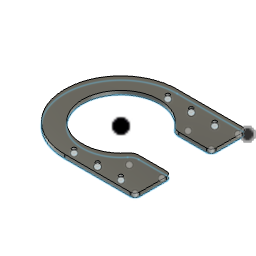
Base (Autodesk Fusion 360 design; units mm, degrees)
Autodesk Fusion 360 part; units mm, degrees
note: some values were not read from the file. Set by a fixed rule: which sketch regions a step uses.
sketch "草图1" plane through (0, 0, 0) normal (0, 0, 1) x (1, 0, 0)
  line L0 (0, 60) -> (70, 60)
  line L1 (75, 55) -> (75, 40)
  line L2 (75, -40) -> (75, -55)
  line L3 (70, -60) -> (0, -60)
  arc A0 (0, 60) -> (0, -60) centre (0, 0) ccw
  circle A1 centre (0, -50) radius 2.1 construction
  circle A2 centre (25, -50) radius 2.1 construction
  circle A3 centre (50, -50) radius 2.1 construction
  circle A4 centre (0, 50) radius 2.1 construction
  circle A5 centre (25, 50) radius 2.1 construction
  circle A6 centre (50, 50) radius 2.1 construction
  circle A7 centre (50, 50) radius 2.1
  circle A8 centre (25, 50) radius 2.1
  circle A9 centre (0, 50) radius 2.1
  circle A10 centre (50, -50) radius 2.1
  circle A11 centre (25, -50) radius 2.1
  circle A12 centre (0, -50) radius 2.1
  arc A13 (32.3364, 25.2063) -> (32.3364, -25.2063) centre (0, 0) ccw
  line L4 (40.2233, 21.3542) -> (70, 21.3542)
  line L5 (75, 26.3542) -> (75, 40)
  line L6 (40.2233, -21.3542) -> (70, -21.3542)
  line L7 (75, -26.3542) -> (75, -40)
  arc A14 (40.2233, -21.3542) -> (32.3364, -25.2063) centre (40.2233, -31.3542) ccw
  arc A15 (32.3364, 25.2063) -> (40.2233, 21.3542) centre (40.2233, 31.3542) ccw
  arc A16 (75, 55) -> (70, 60) centre (70, 55) ccw
  arc A17 (70, 21.3542) -> (75, 26.3542) centre (70, 26.3542) ccw
  arc A18 (75, -26.3542) -> (70, -21.3542) centre (70, -26.3542) ccw
  arc A19 (70, -60) -> (75, -55) centre (70, -55) ccw
  point P0 (75, 60)
  dimension "d2" = 75
  dimension "d41" = 4.2
  dimension "d42" = 4.2
  dimension "d43" = 4.2
  dimension "d44" = 4.2
  dimension "d45" = 4.2
  dimension "d46" = 4.2
  dimension "d55" = 82
  dimension "d56" = 10
  dimension "d57" = 10
  dimension "d58" = 5
  constraint coincident A0.centre A13.centre
  constraint horizontal L0
  constraint vertical L1
  constraint vertical L2
  constraint horizontal L3
  constraint concentric A6 A7
  constraint concentric A5 A8
  constraint concentric A4 A9
  constraint concentric A3 A10
  constraint concentric A2 A11
  constraint concentric A1 A12
  constraint horizontal L4
  constraint vertical L5
  constraint horizontal L6
  constraint vertical L7
  constraint tangent A13 A14
  constraint tangent L6 A14
  constraint tangent A13 A15
  constraint tangent L4 A15
  constraint coincident P0 L0
  constraint coincident P0 L1
  constraint tangent L0 A16
  constraint tangent L1 A16
  constraint tangent L4 A17
  constraint tangent L5 A17
  constraint equal A16 A17
  constraint tangent L6 A18
  constraint tangent L7 A18
  constraint equal A16 A18
  constraint tangent L2 A19
  constraint tangent L3 A19
  constraint equal A16 A19
  measures "d2" distance of L0.start P0
  measures "d41" diameter of A1
  measures "d42" diameter of A2
  measures "d43" diameter of A3
  measures "d44" diameter of A4
  measures "d45" diameter of A5
  measures "d46" diameter of A6
  measures "d55" diameter of A13
  measures "d56" radius of A14
  measures "d57" radius of A15
  measures "d58" radius of A16
extrude "拉伸5" add sketch "草图1" along normal blind 4
extrude "Extrude4" [suppressed]
extrude "Extrude3" [suppressed]
